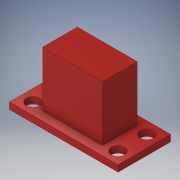
# Autodesk Inventor part: canConnectorModel
Saved by Autodesk Inventor 2018.1 (Build 221171000, 171)
## iProperties
Created: 2017-10-25
Part Number: canConnectorModel
Material: Generic
Document SubType Name: Modeling
Designer: steele
Density: 1 g/cm^3
Appearance: Orange-Red
Author: steele
Autodesk Inventor part; units mm, degrees
ref_plane "YZ Plane" through (0, 0, 0) normal (1, 0, 0) x (0, 1, 0)
ref_plane "XZ Plane" through (0, 0, 0) normal (0, 1, 0) x (-1, 0, 0)
ref_plane "XY Plane" through (0, 0, 0) normal (0, 0, 1) x (1, 0, 0)
sketch "Sketch5" plane through (0, 0, 0) normal (0, 1, 0) x (-1, 0, 0)
  line L0 (13.3477, 6.4516) -> (-13.3477, 6.4516)
  line L1 (-13.3477, 6.4516) -> (-13.3477, -6.4516)
  line L2 (-13.3477, -6.4516) -> (13.3477, -6.4516)
  line L3 (13.3477, -6.4516) -> (13.3477, 6.4516)
  line L4 (13.3477, 6.4516) -> (-13.3477, -6.4516) construction
  line L5 (-13.3477, 6.4516) -> (13.3477, -6.4516) construction
  point P0 (0, 0)
  dimension "d25" = 26.6954
  dimension "d26" = 12.9032
  constraints: 12 end point, 2 midpoint, 2 parallel, 1 horizontal, 1 perpendicular
  measures "d25" distance of L1.end L2.end
  measures "d26" distance of L2.end L0.start
extrude "Extrusion3" add sketch "Sketch5" along normal blind 1.6002
sketch "Sketch6" plane through (0, 1.6002, 0) normal (0, 1, 0) x (1, 0, 0)
  line L0 (-7.3533, -4.2545) -> (7.3533, -4.2545)
  line L1 (7.3533, -4.2545) -> (7.3533, 4.2545)
  line L2 (7.3533, 4.2545) -> (-7.3533, 4.2545)
  line L3 (-7.3533, 4.2545) -> (-7.3533, -4.2545)
  line L4 (-7.3533, -4.2545) -> (7.3533, 4.2545) construction
  line L5 (7.3533, -4.2545) -> (-7.3533, 4.2545) construction
  point P0 (0, 0)
  dimension "d29" = 14.7066
  dimension "d30" = 8.509
  constraints: 12 end point, 2 midpoint, 2 parallel, 1 horizontal, 1 perpendicular
  measures "d29" distance of L1.end L2.end
  measures "d30" distance of L2.end L0.start
extrude "Extrusion4" add sketch "Sketch6" along normal blind 13.589
sketch "Sketch7" plane through (0, 0, 0) normal (0, -1, 0) x (1, 0, 0)
  line L0 (-10.4521, -3.556) -> (10.4521, -3.556) construction
  line L1 (10.4521, -3.556) -> (10.4521, 3.556) construction
  line L2 (10.4521, 3.556) -> (-10.4521, 3.556) construction
  line L3 (-10.4521, 3.556) -> (-10.4521, -3.556) construction
  line L4 (-10.4521, -3.556) -> (10.4521, 3.556) construction
  line L5 (10.4521, -3.556) -> (-10.4521, 3.556) construction
  point P0 (0, 0)
  dimension "d33" = 20.9042
  dimension "d34" = 7.112
  constraints: 12 end point, 4 coincident, 2 midpoint, 2 parallel, 1 horizontal, 1 perpendicular
  measures "d33" distance of L1.end L2.end
  measures "d34" distance of L2.end L0.start
hole "Hole3" at (-10.4521, 0, 3.556) at (10.4521, 0, 3.556) at (10.4521, 0, -3.556) at (-10.4521, 0, -3.556) direction (0, 1, 0) diameter 3.302 end through all
equation "\"d25\" = CanBaseWidth"
equation "\"d26\" = CanBaseLength"
equation "\"d27\" = pcBoardDepth"
equation "\"d29\" = connectorWidth"
equation "\"d30\" = connectorLength"
equation "\"d31\" = connectorHeight"
equation "\"d33\" = HoleWidth"
equation "\"d34\" = HoleLength"
equation "\"CanBaseWidth\" = 26.6954"
equation "\"CanBaseLength\" = 12.9032"
equation "\"HoleWidth\" = 20.9042"
equation "\"HoleLength\" = 7.112"
equation "\"BaseOffset\" = 5.08"
equation "\"PartWidth\" = CanBaseWidth + 2 * BaseOffset"
equation "\"PartLength\" = CanBaseLength + 2 * BaseOffset"
equation "\"boardGap\" = 0.508"
equation "\"boltHeadHeight\" = 3.175"
equation "\"boltHeadDiam\" = 5.08"
equation "\"pcBoardDepth\" = 1.6002"
equation "\"connectorWidth\" = 14.7066"
equation "\"connectorLength\" = 8.509"
equation "\"connectorHeight\" = 13.589"
body "Solid2"
